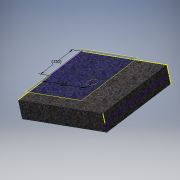
# Autodesk Inventor part: BaseMini
Saved by Autodesk Inventor 2016 (Build 200138000, 138)
## iProperties
Created: 2015-08-01
Part Number: BaseMini
Material: Concrete
Document SubType Name: Modeling
Designer: myhome
Density: 2.40731 g/cm^3
Appearance: Exposed Aggregate - Coarse
Mass: 40442.8 g
Surface Area: 8020 cm^2
Volume: 16800 cm^3
Author: myhome
Autodesk Inventor part; units mm, degrees
ref_plane "YZ Plane" through (0, 0, 0) normal (1, 0, 0) x (0, 1, 0)
ref_plane "XZ Plane" through (0, 0, 0) normal (0, 1, 0) x (-1, 0, 0)
ref_plane "XY Plane" through (0, 0, 0) normal (0, 0, 1) x (1, 0, 0)
sketch "Sketch1" plane through (0, 0, 0) normal (0, 0, 1) x (1, 0, 0)
  line L0 (0, 0) -> (500, 0)
  line L1 (500, 0) -> (500, 500)
  line L2 (500, 500) -> (0, 500)
  line L3 (0, 500) -> (0, 0)
  line L4 (500, 250) -> (0, 250) construction
  line L5 (250, 500) -> (250, 0) construction
  dimension "d0" = 500
  dimension "d1" = 500
  constraints: 12 end point, 4 midpoint, 2 parallel, 1 horizontal, 1 perpendicular
  measures "d0" distance of L1.end L2.end
  measures "d1" distance of L0.end L1.end
extrude "Extrusion1" add sketch "Sketch1" along normal blind 100
sketch "Sketch5" plane through (0, 500, 0) normal (0, 1, 0) x (1, 0, 0)
  line L0 (500, 0) -> (500, -100) projected
  line L1 (500, 0) -> (500, -50)
  line L2 (500, -50) -> (450, -50)
  line L3 (450, -50) -> (400, -50)
  line L4 (400, -50) -> (350, -50)
  line L5 (350, -50) -> (300, -50)
  line L6 (300, -50) -> (250, -50)
  line L7 (250, -50) -> (200, -50)
  line L8 (200, -50) -> (150, -50)
  line L9 (150, -50) -> (0, -50)
  line L10 (0, 0) -> (0, -100) projected
  constraints: 18 end point, 6 point on line, 2 midpoint, 1 horizontal
ref_plane "Work Plane3" through (0, 0, 100) normal (0, 0, -1) x (-1, 0, 0)
sketch "Sketch13" plane through (0, 0, 100) normal (0, 0, -1) x (-1, 0, 0)
  line L0 (0, 500) -> (0, 0) projected
  line L1 (0, 0) -> (-500, 0) projected
  line L2 (0, 0) -> (-250, 0)
  line L3 (-250, 0) -> (-250, 250) construction
  circle A0 centre (-250, 250) radius 27.8669 construction
  dimension "d48" = 250
  dimension "d49" = 250
  constraints: 4 end point, 1 centre point, 1 coincident, 1 midpoint, 1 perpendicular
  measures "d48" distance of L0.end L2.end
  measures "d49" distance of L2.end L3.end
body "Solid1"
